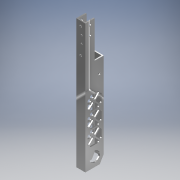
# Autodesk Inventor part: 15102898-16-A-0301
Saved by Autodesk Inventor 2017 (Build 210142000, 142)
## iProperties
Created: 2016-10-02
Part Number: 15102898-16-A-0301
Material: Aluminum 6061
Document SubType Name: Sheet Metal
Designer: gus
Density: 2.7 g/cm^3
Appearance: Aluminum - Flat
Sheet Metal Rule: Default
Mass: 292.173 g
Surface Area: 759.117 cm^2
Volume: 108.212 cm^3
Author: gus
Autodesk Inventor part; units mm, degrees
ref_plane "YZ Plane" through (0, 0, 0) normal (1, 0, 0) x (0, 1, 0)
ref_plane "XZ Plane" through (0, 0, 0) normal (0, 1, 0) x (-1, 0, 0)
ref_plane "XY Plane" through (0, 0, 0) normal (0, 0, 1) x (1, 0, 0)
sketch "Sketch1" plane through (0, 0, 0) normal (0, 1, 0) x (-1, 0, 0)
  line L0 (0, 0) -> (-25.4, 0)
  line L1 (-25.4, 0) -> (-25.4, 50.8)
  line L2 (-25.4, 50.8) -> (0, 50.8)
  line L3 (0, 50.8) -> (0, 0)
  line L4 (-3.175, 3.175) -> (-22.225, 3.175)
  line L5 (-22.225, 3.175) -> (-22.225, 47.625)
  line L6 (-22.225, 47.625) -> (-3.175, 47.625)
  line L7 (-3.175, 47.625) -> (-3.175, 3.175)
  dimension "d0" = 25.4
  dimension "d1" = 50.8
  dimension "d2" = 3.175
  constraints: 16 end point, 4 parallel, 2 perpendicular, 1 horizontal, 3 other
  measures "d0" distance of L1.end L2.end
  measures "d1" distance of L0.end L1.end
  measures "d2" distance between parallel lines of L3 L7
extrude "Extrusion1" add sketch "Sketch1" along normal blind 355.6
sketch "Sketch2" plane through (25.4, 0, 50.8) normal (1, 0, 0) x (0, 0, -1)
  circle A0 centre (25.4, 25.4) radius 14.2875
  line L0 (50.8, 0) -> (50.8, 355.6) projected
  line L1 (50.8, 0) -> (0, 0) projected
  dimension "d5" = 28.575
  dimension "d6" = 25.4
  dimension "d7" = 25.4
  constraints: 1 centre point
  measures "d5" diameter of A0
  measures "d6" distance from line of L0 A0.centre
  measures "d7" distance from line of L1 A0.centre
extrude "Extrusion2" cut sketch "Sketch2" against normal blind 25.4
sketch "Sketch3" plane through (0, 0, 0) normal (-1, 0, 0) x (0, 0, 1)
  line L0 (50.8, 0) -> (50.8, 355.6) projected
  line L1 (0, 355.6) -> (50.8, 355.6) projected
  line L2 (0, 0) -> (0, 355.6) projected
  line L3 (0, 0) -> (50.8, 0) projected
  point P0 (38.1, 346.075)
  point P1 (38.1, 190.5)
  point P2 (38.1, 320.675)
  point P3 (12.7, 215.9)
  dimension "d10" = 12.7
  dimension "d11" = 9.525
  dimension "d19" = 25.4
  dimension "d20" = 38.1
  dimension "d21" = 38.1
  dimension "d23" = 190.5
  dimension "d26" = 215.9
  dimension "d27" = 12.7
  measures "d10" distance from line of L0 point (38.1, 346.075)
  measures "d11" distance from line of L1 point (38.1, 346.075)
  measures "d19" distance of point (38.1, 346.075) point (38.1, 320.675)
  measures "d20" distance from line of L2 point (38.1, 320.675)
  measures "d21" distance from line of L2 point (38.1, 190.5)
  measures "d23" distance from line of L3 point (38.1, 190.5)
  measures "d26" distance from line of L3 point (12.7, 215.9)
  measures "d27" distance from line of point (12.7, 215.9) L2
hole "Hole1" at (0, 346.075, 38.1) at (0, 320.675, 38.1) at (0, 190.5, 38.1) at (0, 215.9, 12.7) direction (1, 0, 0) diameter 6.35 end through all
sketch "Sketch4" plane through (0, 0, 0) normal (-1, 0, 0) x (0, 0, 1)
  line L0 (0, 0) -> (0, 355.6) projected
  line L1 (25.4, 355.6) -> (0, 355.6)
  line L2 (0, 355.6) -> (0, 254)
  line L3 (0, 254) -> (25.4, 254)
  line L4 (25.4, 254) -> (25.4, 355.6)
  line L5 (0, 355.6) -> (50.8, 355.6) projected
  line L6 (50.8, 0) -> (50.8, 355.6) projected
  line L7 (50.8, 0) -> (0, 0) projected
  dimension "d28" = 25.4
  dimension "d29" = 254
  constraints: 8 end point, 2 parallel, 1 collinear, 1 horizontal, 1 perpendicular, 1 point on line
  measures "d28" distance between parallel lines of L6 L4
  measures "d29" distance between parallel lines of L7 L3
extrude "Extrusion3" cut sketch "Sketch4" against normal blind 25.4 contours L0 L1 L4 L3
sketch "Sketch5" plane through (25.4, 0, 50.8) normal (1, 0, 0) x (0, 0, -1)
  line L0 (29.8901, 70.5076) -> (39.4151, 60.9826)
  line L1 (44.8352, 63.2276) -> (44.8352, 82.2776)
  line L2 (39.4151, 84.5227) -> (29.8901, 74.9977)
  line L3 (20.9099, 74.9977) -> (11.3849, 84.5227)
  line L4 (5.9648, 82.2776) -> (5.9648, 63.2276)
  line L5 (0, 0) -> (0, 355.6) projected
  line L6 (11.3849, 60.9826) -> (20.9099, 70.5076)
  line L7 (34.925, 53.3174) -> (15.875, 53.3174)
  line L8 (13.6299, 58.7375) -> (23.1549, 68.2625)
  line L9 (27.6451, 68.2625) -> (37.1701, 58.7375)
  line L10 (27.6451, 77.2428) -> (37.1701, 86.7678)
  line L11 (34.925, 92.1878) -> (15.875, 92.1878)
  line L12 (13.6299, 86.7678) -> (23.1549, 77.2428)
  line L13 (25.4, 74.9977) -> (25.4, 70.5076) construction
  line L14 (27.6451, 72.7526) -> (23.1549, 72.7526) construction
  line L15 (50.8, 0) -> (50.8, 254) projected
  line L16 (44.8352, 89.9428) -> (50.8, 89.9428) construction
  line L17 (5.9648, 89.9428) -> (0, 89.9428) construction
  arc A0 (44.8352, 82.2776) -> (39.4151, 84.5227) centre (41.6602, 82.2776) ccw
  arc A1 (37.1701, 86.7678) -> (34.925, 92.1878) centre (34.925, 89.0128) ccw
  arc A2 (39.4151, 60.9826) -> (44.8352, 63.2276) centre (41.6602, 63.2276) ccw
  arc A3 (29.8901, 74.9977) -> (29.8901, 70.5076) centre (32.1352, 72.7526) ccw
  arc A4 (23.1549, 77.2428) -> (27.6451, 77.2428) centre (25.4, 79.4878) ccw
  arc A5 (15.875, 92.1878) -> (13.6299, 86.7678) centre (15.875, 89.0128) ccw
  arc A6 (34.925, 53.3174) -> (37.1701, 58.7375) centre (34.925, 56.4924) ccw
  arc A7 (27.6451, 68.2625) -> (23.1549, 68.2625) centre (25.4, 66.0174) ccw
  arc A8 (13.6299, 58.7375) -> (15.875, 53.3174) centre (15.875, 56.4924) ccw
  arc A9 (20.9099, 70.5076) -> (20.9099, 74.9977) centre (18.6648, 72.7526) ccw
  arc A10 (5.9648, 63.2276) -> (11.3849, 60.9826) centre (9.1398, 63.2276) ccw
  arc A11 (11.3849, 84.5227) -> (5.9648, 82.2776) centre (9.1398, 82.2776) ccw
  point P0 (44.8352, 55.5625)
  point P1 (5.9648, 55.5625)
  point P2 (8.2099, 53.3174)
  point P3 (42.5901, 53.3174)
  point P4 (42.5901, 92.1878)
  point P5 (8.2099, 92.1878)
  dimension "d35" = 55.5625
  dimension "d39" = 3.175
  dimension "d40" = 3.175
  dimension "d41" = 3.175
  dimension "d50" = 3.175
  dimension "d51" = 19.05
  constraints: 32 end point, 27 point on line, 24 point on circle, 24 tangent, 12 centre point, 11 equal radius, 9 equal length, 5 parallel, 4 perpendicular, 3 horizontal
  measures "d35" vertical distance of L5.start point (5.965, 55.562)
  measures "d39" distance between parallel lines of L12 L3
  measures "d40" distance between parallel lines of L2 L10
  measures "d41" distance between parallel lines of L0 L9
  measures "d50" radius of A0
  measures "d51" distance of A11.centre A10.centre
extrude "Extrusion4" cut sketch "Sketch5" against normal blind 25.4
pattern_linear "Rectangular Pattern1" count 3 spacing 42.0688 along (0, 1, 0) of "Extrusion4"
sketch "Sketch6" plane through (25.4, 0, 50.8) normal (1, 0, 0) x (0, 0, -1)
  line L0 (50.8, 0) -> (50.8, 254) projected
  line L1 (50.8, 19.05) -> (39.8015, 0)
  line L2 (3.175, 0) -> (47.625, 0) projected
  line L3 (50.8, 0) -> (0, 0) projected
  line L4 (47.625, 0) -> (50.8, 0)
  dimension "d52" = 30
  dimension "d53" = 9.525
  constraints: 4 end point, 2 point on line, 1 collinear
  measures "d52" angle of L0 L1
  measures "d53" distance from line of L0.start L1
extrude "Extrusion5" cut sketch "Sketch6" against normal blind 25.4
sketch "Sketch7" plane through (0, 0, 50.8) normal (0, 0, 1) x (1, 0, 0)
  circle A0 centre (12.7, 342.9) radius 3.3782
  circle A1 centre (12.7, 273.05) radius 3.3782
  circle A2 centre (15.24, 322.834) radius 2.5797
  circle A3 centre (15.24, 302.133) radius 2.5797
  line L0 (0, 0) -> (0, 355.6) projected
  line L1 (0, 355.6) -> (25.4, 355.6) projected
  dimension "d56" = 6.7564
  dimension "d57" = 6.7564
  dimension "d58" = 5.1594
  dimension "d59" = 5.1594
  dimension "d60" = 15.24
  dimension "d61" = 15.24
  dimension "d62" = 53.467
  dimension "d63" = 32.766
  dimension "d64" = 12.7
  dimension "d65" = 12.7
  dimension "d66" = 12.7
  dimension "d67" = 82.55
  constraints: 4 centre point
  measures "d56" diameter of A0
  measures "d57" diameter of A1
  measures "d58" diameter of A3
  measures "d59" diameter of A2
  measures "d60" distance from line of L0 A2.centre
  measures "d61" distance from line of L0 A3.centre
  measures "d62" distance from line of L1 A3.centre
  measures "d63" distance from line of L1 A2.centre
  measures "d64" distance from line of L1 A0.centre
  measures "d65" distance from line of L0 A0.centre
  measures "d66" distance from line of L0 A1.centre
  measures "d67" distance from line of L1 A1.centre
extrude "Extrusion6" cut sketch "Sketch7" against normal blind 25.4
equation "\"BendRadius\" = Thickness"
equation "\"BendReliefWidth\" = Thickness"
equation "\"BendReliefDepth\" = 0.5 * Thickness"
equation "\"CornerReliefSize\" = 4 * Thickness"
equation "\"MinimumRemnant\" = 2 * Thickness"
equation "\"TransitionRadius\" = BendRadius"
equation "\"JacobiRadiusSize\" = Thickness"
equation "\"GapSize\" = Thickness"
equation "\"Thickness\" = 3.048"
body "Solid1"
